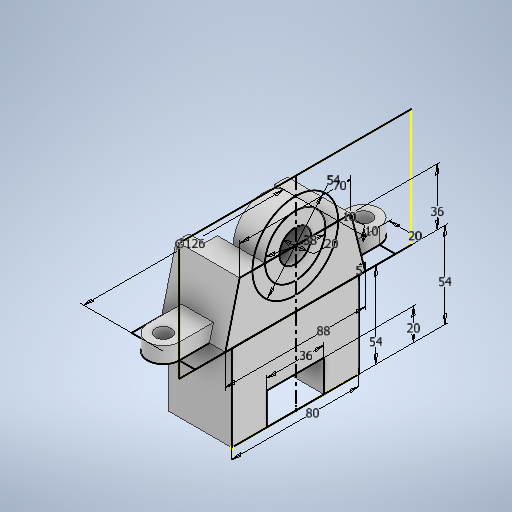
# Autodesk Inventor part: Baitap3
Saved by Autodesk Inventor 2025.2 (Build 292293000, 293)
## iProperties
Created: 2024-12-04
Part Number: Baitap3
Material: Generic
Document SubType Name: Modeling
Designer: hongquan
Density: 1 g/cm^3
Appearance: Default
Author: hongquan
Autodesk Inventor part; units mm, degrees
ref_plane "YZ Plane" through (0, 0, 0) normal (1, 0, 0) x (0, 1, 0)
ref_plane "XZ Plane" through (0, 0, 0) normal (0, 1, 0) x (-1, 0, 0)
ref_plane "XY Plane" through (0, 0, 0) normal (0, 0, 1) x (1, 0, 0)
sketch "Sketch1" plane through (0, 0, 0) normal (1, 0, 0) x (0, 1, 0)
  line L0 (0, 0) -> (54, 0)
  line L1 (54, 0) -> (54, -80)
  line L2 (54, -80) -> (0, -80)
  line L3 (0, -80) -> (0, 0)
  dimension "d0" = 80
  dimension "d1" = 54
  constraints: 8 end point, 2 parallel, 1 horizontal, 1 perpendicular
  measures "d0" distance of L2.end L0.start
  measures "d1" distance of L1.end L2.end
extrude "Extrusion1" add sketch "Sketch1" against normal blind 40
sketch "Sketch2" plane through (0, 0, 0) normal (1, 0, 0) x (0, 0, -1)
  line L0 (22, 20) -> (58, 20)
  line L1 (0, 0) -> (80, 0) projected
  line L2 (0, 54) -> (80, 54) projected
  line L3 (40, 54) -> (40, 0)
  line L4 (22, 20) -> (22, 0)
  line L5 (58, 20) -> (58, 0)
  line L6 (22, 0) -> (58, 0)
  line L7 (80, 0) -> (0, 0) projected
  point P0 (40, 20)
  dimension "d4" = 36
  dimension "d5" = 20
  constraints: 10 end point, 3 midpoint, 3 point on line, 2 perpendicular, 1 collinear, 1 horizontal
  measures "d4" distance of L0.start L0.end
  measures "d5" distance between parallel lines of L1 L0
extrude "Extrusion2" cut sketch "Sketch2" against normal blind 40
sketch "Sketch3" plane through (0, 54, 0) normal (0, 1, 0) x (1, 0, 0)
  line L0 (-40, 58) -> (-40, 22) projected
  line L1 (-40, 40) -> (0, 40)
  line L2 (0, 22) -> (0, 58) projected
  line L3 (0, 0) -> (-40, 0) projected
  line L4 (-20, 0) -> (-20, 80) construction
  line L5 (0, 80) -> (-40, 80) projected
  circle A0 centre (-20, 103) radius 5
  arc A1 (-10, 103) -> (-30, 103) centre (-20, 103) ccw
  line L6 (-40, 40) -> (-40, 103)
  line L7 (-40, 103) -> (-30, 103)
  line L8 (0, 40) -> (0, 103)
  line L9 (0, 103) -> (-10, 103)
  circle A2 centre (-20, -23) radius 5
  arc A3 (-30, -23) -> (-10, -23) centre (-20, -23) ccw
  line L10 (-40, 40) -> (-40, -23)
  line L11 (-40, -23) -> (-30, -23)
  line L12 (0, 40) -> (0, -23)
  line L13 (0, -23) -> (-10, -23)
  line L14 (-10, 103) -> (-10, -23)
  line L15 (-30, 103) -> (-30, -23)
  point P0 (-10, 0)
  point P1 (-30, 0)
  point P2 (-30, 80)
  point P3 (-10, 80)
  dimension "d8" = 10
  dimension "d9" = 20
  dimension "d10" = 126
  dimension "d11" = 10
  constraints: 24 end point, 6 symmetric about line, 5 point on circle, 4 centre point, 4 midpoint, 2 coincident, 2 perpendicular, 2 vertical, 1 horizontal, 1 parallel, 1 point on line, 1 tangent, 2 other
  measures "d8" diameter of A0
  measures "d9" distance from line of L2 A0.centre
  measures "d10" diameter of A0.centre L1
  measures "d11" radius of A1
extrude "Extrusion3" add sketch "Sketch3" along normal blind 74
sketch "Sketch4" plane through (0, 0, 0) normal (1, 0, 0) x (0, 0, -1)
  line L0 (-4, 54) -> (84, 54)
  line L1 (-23, 128) -> (103, 128) projected
  line L2 (40, 128) -> (40, 0)
  line L3 (58, 0) -> (80, 0) projected
  line L4 (84, 54) -> (84, 59)
  circle A0 centre (40, 90) radius 19
  circle A1 centre (40, 90) radius 10
  circle A2 centre (40, 90) radius 27
  line L5 (5, 90) -> (75, 90)
  line L6 (5, 90) -> (-4, 54)
  line L7 (75, 90) -> (84, 54)
  line L8 (-23, 54) -> (-33, 54) projected
  line L9 (113, 54) -> (113, 128) projected
  line L10 (113, 54) -> (103, 54) projected
  line L11 (-33, 54) -> (113, 54)
  line L12 (-23, 128) -> (-33, 128) projected
  line L13 (-33, 128) -> (113, 128)
  line L14 (-33, 128) -> (-33, 54)
  line L15 (-33, 54) -> (-33, 128) projected
  line L16 (13, 90) -> (67, 90)
  line L17 (13, 90) -> (67, 90)
  point P0 (0, 0)
  point P1 (40, 54)
  point P2 (59, 90)
  point P3 (21, 90)
  point P4 (30, 90)
  point P5 (50, 90)
  dimension "d14" = 88
  dimension "d15" = 54
  dimension "d16" = 5
  dimension "d17" = 38
  dimension "d18" = 20
  dimension "d22" = 70
  dimension "d23" = 36
  dimension "d28" = 54
  constraints: 22 end point, 4 collinear, 4 midpoint, 4 point on line, 3 centre point, 2 coincident, 2 horizontal, 2 point on circle, 2 vertical
  measures "d14" distance of L0.start L0.end
  measures "d15" distance between parallel lines of L3 L0
  measures "d16" distance of L0.end L4.end
  measures "d17" diameter of A0
  measures "d18" diameter of A1
  measures "d22" distance of L5.start L5.end
  measures "d23" distance of point (40, 54) A0.centre
  measures "d28" diameter of A2
extrude "Extrusion4" cut sketch "Sketch4" against normal blind 74 contours L11 L8 L14 L12 L1 L2 A2 L5 L6 | L7 L5 A2 L2 L1 L13 L9 L10 L11
extrude "Extrusion5" cut sketch "Sketch4" against normal blind 74 contours A2 L5 A0 L2 | L2 A0 L5 A2 | A2 L2 A0 L5 | A0 L5 A1 L2 | L2 A1 L5 A0 | L5 A0 L2 A2 | A0 L2 A1 L5 | A1 L5 L2 | L2 L5 A1 | L5 A1 L2 A0 | A1 L2 L5 | L2 A1 L5
extrude "Extrusion6" add sketch "Sketch4" against normal blind 30 contours A2 L5 A0 L2 | L2 A0 L5 A2 picked at (15.8923, 87.9973) picked at (64.1077, 87.9973)
extrude "Extrusion7" add sketch "Sketch4" against normal blind 20 contours A0 L5 A1 L2 | L2 A1 L5 A0 picked at (24.1588, 88.5907) picked at (55.7576, 87.849)
extrude "Extrusion8" add sketch "Sketch4" against normal blind 20 contours A0 L2 A1 L5 | L5 A1 L2 A0 picked at (24.8696, 94.899) picked at (53.2638, 98.775)
extrude "Extrusion9" add sketch "Sketch3" along normal blind 10 contours L15 A1 L14 L5 | L3 L14 A3 L15
body "Solid1"
